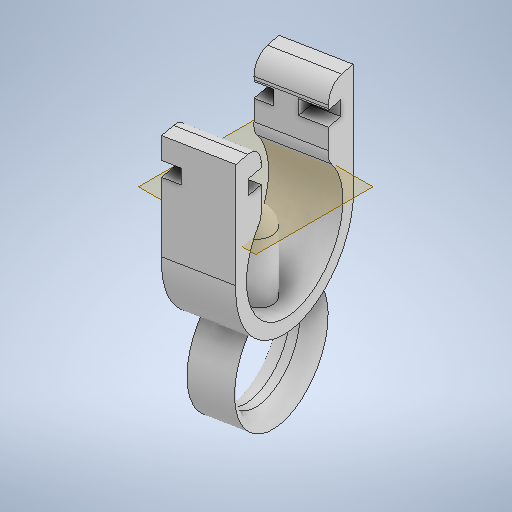
# Autodesk Inventor part: Clip8
Saved by Autodesk Inventor 2025 (Build 290162010, 162A)
## iProperties
Created: 2026-02-19
Part Number: Clip8
Material: Generic
Document SubType Name: Modeling
Designer: 925699
Density: 1 g/cm^3
Appearance: Default
Author: 925699
Autodesk Inventor part; units mm, degrees
ref_plane "YZ Plane" through (0, 0, 0) normal (1, 0, 0) x (0, 1, 0)
sketch "Sketch1" plane through (0, 0, 0) normal (0, 0, 1) x (1, 0, 0)
  line L0 (0, 0) -> (0, 15.1122)
  line L1 (3.0357, 11.4778) -> (3.0357, 0)
  line L2 (3.0357, 0) -> (0, 0)
  arc A0 (3.0357, 11.4778) -> (0, 15.1122) centre (-0.6577, 11.4778) ccw
  constraints: 6 end point, 2 point on circle, 1 centre point, 1 horizontal, 1 tangent
ref_plane "Work Plane3" through (0, 17.8837, 0) normal (0, 1, 0) x (1, 0, 0)
ref_plane "Work Plane1" through (-3.9896, 4.3483, 0.7741) normal (-0.9816919, 0, 0.1904757) x (0, -1, 0)
sketch "Sketch3" plane through (-3.9896, 4.3483, 0.7741) normal (-0.9816919, 0, 0.1904757) x (0, -1, 0)
  arc A0 (-16.337, -6.8791) -> (-16.337, 6.8791) centre (-7.2089, 0) ccw
  arc A1 (-18.3655, -8.4078) -> (-18.3655, 8.4078) centre (-7.2089, 0) ccw
  line L0 (-13.5354, -0.5887) -> (0.7521, -0.5887) projected
  line L1 (-13.5354, 0.6171) -> (0.7521, 0.6171) projected
  line L2 (-7.2089, 0) -> (-7.9901, -0.5887)
  line L3 (-16.337, -6.8791) -> (-18.3655, -8.4078)
  line L4 (-7.2089, 0) -> (-8.0277, 0.6171)
  line L5 (-16.337, 6.8791) -> (-18.3655, 8.4078)
  constraints: 8 end point, 4 point on circle, 2 centre point, 2 coincident, 2 point on line
extrude "Extrusion2" add sketch "Sketch3" along normal blind 1.5875 and the other way blind 10.3124
fillet "Fillet1" radius 3.175 2 edges at (-1.0173, 20.6854, -6.81) (1.6033, 20.6854, 6.6963)
ref_plane "Work Plane2" through (0.293, 4.3483, -0.0568) normal (0.9816919, 0, -0.1904757) x (-0.1904757, 0, -0.9816919)
sketch "Sketch4" plane through (0.293, 4.3483, -0.0568) normal (0.9816919, 0, -0.1904757) x (-0.1904757, 0, -0.9816919)
  circle A0 centre (0, -12.1867) radius 8.89
  arc A1 (-8.4078, 18.3655) -> (8.4078, 18.3655) centre (0, 7.2089) ccw projected
  arc A2 (-7.848, -4.3483) -> (7.848, -4.3483) centre (0, -12.1867) ccw
  point P0 (0, -4.3483)
  point P1 (5.8384, -5.4826)
  point P2 (-5.8384, -5.4826)
  dimension "d17" = 17.78
  constraints: 4 point on circle, 2 centre point, 1 concentric
  measures "d17" diameter of A0
extrude "Extrusion3" add sketch "Sketch4" along normal mid plane 7.62 contours A0 A1 A2
fillet "Fillet2" radius 3.175 2 edges at (-3.4473, -16.7283, 0.6689) (4.0332, -16.7283, -0.7826)
sketch "Sketch5" plane through (-5.548, 4.3483, 1.0765) normal (-0.9816919, 0, 0.1904757) x (0.1904757, 0, 0.9816919)
  arc A0 (-8.6921, 14.6313) -> (-8.4078, 18.3655) centre (-11.1066, 16.6931) ccw projected
  line L0 (-7.9735, 17.2071) -> (-7.9735, 24.0368)
  line L1 (-10.116, 16.8437) -> (-10.116, 16.3667)
  arc A1 (8.4078, 18.3655) -> (8.6921, 14.6313) centre (11.1066, 16.6931) ccw projected
  line L2 (7.9735, 17.2071) -> (7.9735, 24.0368)
  line L3 (10.0556, 16.9067) -> (10.0556, 16.0648)
  line L4 (-8.0331, 17.1837) -> (-7.9735, 17.2071)
  line L5 (-7.9735, 24.0368) -> (-7.9408, 27.7976)
  line L6 (-10.116, 27.7976) -> (-7.9408, 27.7976)
  line L7 (7.9408, 27.7976) -> (10.0556, 27.7976)
  arc A2 (-8.4078, 18.3655) -> (8.4078, 18.3655) centre (0, 7.2089) ccw projected
  line L8 (7.9408, 27.7976) -> (13.9423, 27.7976)
  line L9 (13.9423, 27.7976) -> (13.9423, 6.3292)
  line L10 (13.9423, 6.3292) -> (13.9416, 6.3292)
  line L11 (7.9408, 16.452) -> (7.9408, 27.7976)
  line L12 (-7.9408, 27.7976) -> (-13.876, 27.7976)
  line L13 (-13.876, 27.7976) -> (-13.876, 6.3292)
  line L14 (-7.9408, 16.452) -> (-7.9408, 27.7976)
  arc A3 (13.9421, 6.3267) -> (7.9408, 16.452) centre (-4.3172, 2.3454) ccw
  arc A4 (-7.9408, 16.452) -> (-13.876, 6.3292) centre (3.6251, 2.8693) ccw
  line L15 (-8.1275, 6.3292) -> (-7.9408, 6.3292)
  point P0 (0, -4.3483)
  point P1 (10.0556, 24.2784)
  point P2 (7.9735, 31.5584)
  point P3 (-7.9735, 31.5584)
  point P4 (-10.116, 31.5584)
  point P5 (-10.116, 27.7976)
  point P6 (-13.876, 8.8266)
  point P7 (7.9408, 16.9341)
  point P8 (13.9423, 8.0887)
  point P9 (10.0556, 27.7976)
  constraints: 32 end point, 14 point on circle, 6 point on line, 4 parallel, 2 centre point, 2 horizontal, 2 perpendicular, 2 vertical
sketch "Sketch6" plane through (-5.548, 4.3483, 1.0765) normal (-0.9816919, 0, 0.1904757) x (0.1904757, 0, 0.9816919)
  line L0 (11.5164, 23.7535) -> (-13.6635, 23.7535)
  line L1 (-13.6635, 21.0208) -> (11.5164, 21.0208)
  line L2 (-26.4342, 23.7535) -> (27.1088, 23.7535)
  line L3 (27.1088, 23.7535) -> (27.1088, 21.0208)
  line L4 (27.1088, 21.0208) -> (-26.4342, 21.0208)
  line L5 (-26.4342, 21.0208) -> (-26.4342, 23.7535)
  point P0 (0, -4.3483)
  point P1 (11.5164, 23.7535)
  point P2 (-13.6635, 21.0208)
  constraints: 12 end point, 3 parallel, 2 horizontal, 1 perpendicular, 1 point on line
revolve "Revolution3" add sketch "Sketch1" angle 360 about axis through (0, 0, 0) along (0, 1, 0)
extrude "Extrusion7" add sketch "Sketch5" against normal up to surface (11.8999 mm away) contours A0 A2 L13 L12 L6 L5 L0 | A1 L11 L7 L8 L9 A2
extrude "Extrusion8" cut sketch "Sketch6" against normal blind 3.175
fillet "Fillet4" radius 3.175 2 edges at (-1.2195, 32.1459, -7.8522) (1.8055, 32.1459, 7.7386)
sketch "Sketch8" plane through (6.134, 4.3483, -1.1902) normal (0.9816919, 0, -0.1904757) x (-0.1904757, 0, -0.9816919)
  line L0 (-13.9423, 21.0208) -> (-7.9408, 21.0208) projected
  line L1 (-7.9408, 23.7535) -> (-13.9423, 23.7535) projected
  line L2 (-7.9408, 21.0208) -> (-10.9415, 21.0208)
  line L3 (-10.9415, 21.0208) -> (-10.9415, 23.7535)
  line L4 (-10.9415, 23.7535) -> (-7.9408, 23.7535)
  line L5 (-7.9408, 23.7535) -> (-7.9408, 21.0208)
  line L6 (7.9408, 21.0208) -> (10.9415, 21.0208)
  line L7 (10.9415, 21.0208) -> (10.9415, 23.7535)
  line L8 (10.9415, 23.7535) -> (7.9408, 23.7535)
  line L9 (7.9408, 23.7535) -> (7.9408, 21.0208)
  point P0 (0, -4.3483)
  point P1 (7.9408, 23.7535)
  point P2 (-7.9408, 23.7535)
  point P3 (-10.9415, 21.0208)
  constraints: 16 end point, 2 parallel, 1 horizontal, 1 midpoint, 1 perpendicular
extrude "Extrusion9" cut sketch "Sketch8" against normal blind 4.7625
body "Solid1"
